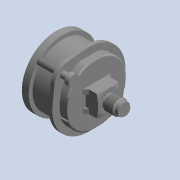
# Autodesk Inventor part: Vacuometro1
Saved by Autodesk Inventor 2021 (Build 250183000, 183)
## iProperties
Category: PARTsolutions
Company: FESTO
Part Number: Vacuometro1
Material: Genérico
Catalog Web Link: www.cadenas.de
Description: FVAM-vacuum gauge
Vendor: FESTO
Document SubType Name: Modeling
Designer: partserver
Manufacturer: FESTO
Mass: 81 g
Surface Area: 95.1395 cm^2
Volume: 38.5527 cm^3
Density: 1 g/cm^3
Appearance: PSOLRGB-175-175-175
PSOL_IDENT_0: {$CADENAS_DATA\23d-libs\festo\parts\f\fvam\fvam.prj},192 {VTYP=3D},{NB=537812 FVAM-40-V1/0-G1/8-EN},
PSOL_IDENT_1: {LINA=537812 FVAM-40-V1/0-G1/8-EN},{NN=FVAM},{DATE=03.03.2020 11:57:51},{GEOMDATE=02.03.2020 14:51:1
PSOL_IDENT_2: 6},{VERSION=},{LINEID=20},{WBVAR=},{WBNUMERIC=}  {NB=537812 FVAM-40-V1/0-G1/8-EN},{LINA=537812 FVAM-
PSOL_IDENT_3: 40-V1/0-G1/8-EN},{KT=DUMMY},{TNR=537812},{TYP=FVAM-40-V1/0-G1/8-EN},{VERS=1.000},{CNSMASSEXACT=0.081
PSOL_IDENT_4: }
NB: 537812 FVAM-40-V1/0-G1/8-EN
NN: FVAM
NT: vacuum gauge
NBSYN: $TNR. $TYP.
LINA: 537812 FVAM-40-V1/0-G1/8-EN
CATALOG: Festo
TNR: 537812
TYP: FVAM-40-V1/0-G1/8-EN
CNSMASSEXACT: 0.081
SUPPLIER: FESTO
ARTICLENO: 537812 FVAM-40-V1/0-G1/8-EN
BOMINFO: 537812 FVAM-40-V1/0-G1/8-EN
CREATOR: CADENAS GmbH
Title: 537812 FVAM-40-V1/0-G1/8-EN
Author: Cadenas PARTsolutions
Comments: vacuum gauge
Autodesk Inventor part; units mm, degrees
sketch "Skizze_1" plane through (0, 0, 0) normal (0, 0, 1) x (1, 0, 0)
  line L0 (34.5, 0) -> (-10, 0)
  line L1 (8, 0) -> (8, 19)
  arc A0 (9, 20) -> (8, 19) centre (9, 19) ccw
  line L2 (9, 20) -> (30, 20)
  line L3 (30, 20) -> (30, 22.5)
  line L4 (30, 22.5) -> (34.5, 22.5)
  line L5 (34.5, 22.5) -> (34.5, 19.65)
  arc A1 (34.2, 19.35) -> (34.5, 19.65) centre (34.2, 19.65) ccw
  line L6 (34.2, 19.35) -> (34, 19.35)
  line L7 (34, 19.35) -> (34, 0)
  line L8 (34, 0) -> (8, 0)
  constraints: 18 end point, 4 point on circle, 2 centre point
revolve "Revolution1" add sketch "Skizze_1" angle 360 about axis through (34.5, 0, 0) along (1, 0, 0)
sketch "Skizze_2" plane through (0, 0, 0) normal (1, 0, 0) x (0, 1, 0)
  line L0 (-7, 7) -> (-7, -7)
  line L1 (-7, -7) -> (7, -7)
  line L2 (7, -7) -> (7, 7)
  line L3 (7, 7) -> (-7, 7)
  constraints: 8 end point
extrude "Extrusion1" add sketch "Skizze_2" along normal blind 10
sketch "Skizze_3" plane through (0, 0, 0) normal (0, 0, 1) x (1, 0, 0)
  line L0 (5, 0) -> (-5, 0)
  arc A0 (1, 10) -> (0, 7) centre (7.9398, 6.0201) ccw
  line L1 (1, 10) -> (1, 17)
  line L2 (1, 17) -> (0, 17)
  line L3 (0, 17) -> (0, 7)
  constraints: 8 end point, 2 point on circle, 1 centre point
revolve "Revolution2" cut sketch "Skizze_3" angle 360 about axis through (5, 0, 0) along (1, 0, 0)
sketch "Skizze_6" plane through (8, 0, 0) normal (1, 0, 0) x (0, 0, -1)
  line L0 (-5, 29) -> (-5, 19)
  line L1 (-5, 19) -> (-3.0923, 19)
  arc A0 (3.0923, 19) -> (-3.0923, 19) centre (0, 0) ccw
  line L2 (3.0923, 19) -> (5, 19)
  line L3 (5, 19) -> (5, 29)
  line L4 (5, 29) -> (-5, 29)
  constraints: 10 end point, 2 point on circle, 1 centre point
extrude "Extrusion2" cut sketch "Skizze_6" along normal blind 5
sketch "Skizze_4" plane through (0, 0, 0) normal (0, 0, 1) x (1, 0, 0)
  line L0 (50, 0) -> (-50, 0)
  line L1 (13, 29.25) -> (13, 19.25)
  line L2 (13, 19.25) -> (15.5, 19.25)
  line L3 (15.5, 19.25) -> (25.5, 29.25)
  line L4 (25.5, 29.25) -> (13, 29.25)
  constraints: 10 end point
revolve "Revolution3" cut sketch "Skizze_4" angle 148.6 mid plane about axis through (50, 0, 0) along (-1, 0, 0)
sketch "Skizze_5" plane through (0, 0, 0) normal (0, 0, 1) x (1, 0, 0)
  line L0 (-50, 0) -> (50, 0)
  line L1 (8, -29.25) -> (25.5, -29.25)
  line L2 (25.5, -29.25) -> (15.5, -19.25)
  line L3 (15.5, -19.25) -> (8, -19.25)
  line L4 (8, -19.25) -> (8, -29.25)
  constraints: 10 end point
revolve "Revolution4" cut sketch "Skizze_5" angle 40 mid plane about axis through (-50, 0, 0) along (1, 0, 0)
sketch "Skizze_7" plane through (8, 0, 0) normal (1, 0, 0) x (0, 0, -1)
  line L0 (-30, -40) -> (30, -40)
  line L1 (30, -40) -> (30, 40)
  line L2 (30, 40) -> (-30, 40)
  line L3 (-30, 40) -> (-30, -40)
  line L4 (-19, -25) -> (19, -25)
  line L5 (19, -25) -> (19, 25)
  line L6 (19, 25) -> (-19, 25)
  line L7 (-19, 25) -> (-19, -25)
  constraints: 16 end point
extrude "Extrusion3" cut sketch "Skizze_7" along normal blind 8.2
sketch "Skizze_8" plane through (0, 0, 7) normal (0, 0, 1) x (1, 0, 0)
  line L0 (6, -7) -> (8, -9)
  line L1 (8, -9) -> (8, 9)
  line L2 (8, 9) -> (6, 7)
  line L3 (6, 7) -> (6, -7)
  constraints: 8 end point
extrude "Extrusion4" add sketch "Skizze_8" against normal blind 3
sketch "Skizze_9" plane through (0, 0, -7) normal (0, 0, 1) x (1, 0, 0)
  line L0 (6, -7) -> (8, -9)
  line L1 (8, -9) -> (8, 9)
  line L2 (8, 9) -> (6, 7)
  line L3 (6, 7) -> (6, -7)
  constraints: 8 end point
extrude "Extrusion5" add sketch "Skizze_9" along normal blind 3
sketch "Skizze_11" plane through (13, 0, 0) normal (1, 0, 0) x (0, 0, -1)
  arc A0 (-23.866, 2.5327) -> (2.5327, -23.866) centre (0, 0) ccw
  line L0 (2.5327, -23.866) -> (13.7832, -22.6721)
  arc A1 (13.7832, -22.6721) -> (22.6721, -13.7832) centre (12.7279, -12.7279) ccw
  line L1 (22.6721, -13.7832) -> (23.866, -2.5327)
  arc A2 (23.866, -2.5327) -> (-2.5327, 23.866) centre (0, 0) ccw
  line L2 (-2.5327, 23.866) -> (-13.7832, 22.6721)
  arc A3 (-13.7832, 22.6721) -> (-22.6721, 13.7832) centre (-12.7279, 12.7279) ccw
  line L3 (-22.6721, 13.7832) -> (-23.866, 2.5327)
  constraints: 8 end point, 8 point on circle, 4 centre point
extrude "Extrusion6" add sketch "Skizze_11" along normal blind 2.5
sketch "Skizze_12" plane through (0, 0, 0) normal (0, -0.7071068, 0.7071068) x (1, 0, 0)
  line L0 (28.6, 24) -> (6, 24)
  line L1 (6, 24) -> (6, 27.2725)
  line L2 (6, 27.2725) -> (8.6, 27.5)
  line L3 (8.6, 27.5) -> (8.6, 26)
  line L4 (8.6, 26) -> (28.1705, 26)
  line L5 (28.1705, 26) -> (28.6, 25.5705)
  line L6 (28.6, 25.5705) -> (28.6, 24)
  line L7 (28.6, 24) -> (6, 24)
  constraints: 16 end point
revolve "Revolution5" add sketch "Skizze_12" angle 360 about axis through (28.6, 16.9706, 16.9706) along (1, 0, 0)
thread "Thread1" size "M4x0.7" class "6g" standard "ISO Metric profile" length 18.5705
sketch "Skizze_13" plane through (0, 0, 0) normal (0, -0.7071068, 0.7071068) x (1, 0, 0)
  line L0 (28.6, -24) -> (6, -24)
  line L1 (6, -24) -> (6, -20.7275)
  line L2 (6, -20.7275) -> (8.6, -20.5)
  line L3 (8.6, -20.5) -> (8.6, -22)
  line L4 (8.6, -22) -> (28.1705, -22)
  line L5 (28.1705, -22) -> (28.6, -22.4295)
  line L6 (28.6, -22.4295) -> (28.6, -24)
  line L7 (28.6, -24) -> (6, -24)
  constraints: 16 end point
revolve "Revolution6" add sketch "Skizze_13" angle 360 about axis through (28.6, -16.9706, -16.9706) along (1, 0, 0)
thread "Thread2" size "M4x0.7" class "6g" standard "ISO Metric profile" length 18.5705
sketch "Skizze_10" plane through (0, 0, 0) normal (0, 0, 1) x (1, 0, 0)
  line L0 (0, 0) -> (-10, 0)
  line L1 (-10, 0) -> (-10, 4)
  line L2 (-10, 4) -> (-8, 4)
  line L3 (-8, 4) -> (-8, 4.283)
  line L4 (-8, 4.283) -> (-7.419, 4.864)
  line L5 (-7.419, 4.864) -> (-1.5, 4.864)
  line L6 (-1.5, 4.864) -> (-1.1455, 4.25)
  arc A0 (-1.1455, 4.25) -> (-0.7125, 4) centre (-0.7125, 4.5) ccw
  line L7 (-0.7125, 4) -> (-0.3, 4)
  arc A1 (-0.3, 4) -> (0, 4.3) centre (-0.3, 4.3) ccw
  line L8 (0, 4.3) -> (0, 0)
  line L9 (0, 0) -> (-10, 0)
  constraints: 20 end point, 4 point on circle, 2 centre point
revolve "Revolution7" add sketch "Skizze_10" angle 360 about axis through (0, 0, 0) along (1, 0, 0)
thread "Thread3" size "G9.728x0.907" designation "G 1/8" class "A" standard "ISO Pipe Threads" full length
ref_plane "ANBAU_XY" through (0, 0, 0) normal (1, 0, 0) x (0, 0, -1)
ref_plane "ANBAU_YZ" through (0, 0, 0) normal (0, 0, -1) x (0, 1, 0)
ref_plane "ANBAU_ZX" through (0, 0, 0) normal (0, 1, 0) x (1, 0, 0)
body "Solid1"
